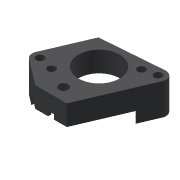
# Autodesk Inventor part: linact_top
Saved by Autodesk Inventor 2014 (Build 180170000, 170)
## iProperties
Created: 2015-04-17
Part Number: linact_top
Material: Generic
Document SubType Name: Modeling
Designer: Martin
Density: 1 g/cm^3
Appearance: Default
Mass: 1.23185 g
Surface Area: 12.9217 cm^2
Volume: 1.23185 cm^3
Author: Martin
Autodesk Inventor part; units mm, degrees
sketch "sk_mainbody" plane through (0, 0, 0) normal (0, 0, 1) x (1, 0, 0)
  line L0 (-7.1386, -0.6138) -> (9.4827, 3.383) construction
  line L1 (-10.6899, -8.9546) -> (-7.1386, -0.6138) projected
  arc A0 (-10.6899, -8.9546) -> (-10.0592, -11.3309) centre (-8.8497, -9.7381) ccw projected
  line L2 (-3.4497, -16.3498) -> (-10.0592, -11.3309) projected
  circle A1 centre (-8.8497, -9.7381) radius 1 projected
  circle A2 centre (9.9503, 1.4384) radius 1 projected
  arc A3 (11.7904, 0.655) -> (9.4827, 3.383) centre (9.9503, 1.4384) ccw projected
  line L3 (11.7904, 0.655) -> (4.5503, -16.3498) projected
  line L4 (4.5503, -16.3498) -> (-3.4497, -16.3498) projected
  circle A4 centre (0.5503, -4.1498) radius 3.4 construction
  circle A5 centre (0.5503, -13.1498) radius 1 construction
  circle A6 centre (0.5503, -4.1498) radius 5.25
  line L5 (-7.1386, -0.6138) -> (-5.9457, 2.1878)
  line L6 (-5.9457, 2.1878) -> (9.7927, 3.4322)
  circle A7 centre (0.5503, -13.1498) radius 1.2
  point P0 (0, 0)
  dimension "d0" = 10.5
  dimension "d1" = 9
  dimension "d37" = 2.4
  constraints: 4 end point, 2 centre point, 2 coincident, 1 parallel, 1 point on circle, 1 tangent
  measures "d0" diameter of A6
  measures "d1" angle of L0 L6
  measures "d37" diameter of A7
extrude "ext_mainbody" add sketch "sk_mainbody" along normal blind 5.2
sketch "sk_bottomsupport" plane through (0, 0, 0) normal (0, 0, 1) x (1, 0, 0)
  line L0 (-10.6899, -8.9546) -> (-7.1386, -0.6138) projected
  arc A0 (-10.6899, -8.9546) -> (-10.0592, -11.3309) centre (-8.8497, -9.7381) ccw projected
  line L1 (-3.4497, -16.3498) -> (-10.0592, -11.3309) projected
  line L2 (4.5503, -16.3498) -> (-3.4497, -16.3498) projected
  line L3 (11.7904, 0.655) -> (4.5503, -16.3498) projected
  arc A1 (11.7904, 0.655) -> (9.4827, 3.383) centre (9.9503, 1.4384) ccw projected
  line L4 (-7.1386, -0.6138) -> (9.4827, 3.383) projected
  circle A2 centre (-8.8497, -9.7381) radius 1 projected
  circle A3 centre (9.9503, 1.4384) radius 1 projected
  circle A4 centre (0.5503, -13.1498) radius 1 construction
  arc A5 (-6.417, -9.0187) -> (-7.5492, -13.2368) centre (0.5503, -13.1498) ccw
  circle A6 centre (-4.5247, -4.1498) radius 1 construction
  circle A7 centre (0.5503, -4.1498) radius 3.4 construction
  circle A8 centre (0.5503, -4.1498) radius 5 construction
  circle A9 centre (-5.0196, -10.6625) radius 2 construction
  circle A10 centre (6.5473, 0.6202) radius 2 construction
  circle A11 centre (6.5473, 0.6202) radius 1
  circle A12 centre (-5.0196, -10.6625) radius 1
  circle A13 centre (9.9503, 1.4384) radius 1.5 construction
  circle A14 centre (0.5503, -4.1498) radius 5.6627 construction
  arc A15 (-7.9094, -4.9768) -> (-6.417, -9.0187) centre (0.5503, -4.1498) ccw
  line L5 (-7.9094, -4.9768) -> (-8.8294, -4.5851)
  line L6 (8.0243, 3.0323) -> (8.4919, 1.0877)
  arc A16 (7.9873, -0.7678) -> (8.4919, 1.0877) centre (6.5473, 0.6202) ccw
  line L7 (-5.0196, -10.6625) -> (-7.1846, -13.5137) construction
  line L8 (-5.0196, -10.6625) -> (-2.8545, -7.8114) construction
  line L9 (7.9873, -0.7678) -> (9.7823, -4.0616)
  arc A17 (8.2936, -0.3548) -> (8.2887, -1.3207) centre (9.1667, -0.8422) ccw
  line L10 (9.7927, 3.4322) -> (-5.9457, 2.1878) projected
  line L11 (8.0243, 3.0323) -> (7.9629, 3.2876)
  point P0 (0, 0)
  point P1 (-5.2757, -0.1658)
  dimension "d12" = 10
  dimension "d16" = 3
  dimension "d5" = 8.1
  dimension "d13" = 4
  dimension "d15" = 2
  dimension "d17" = 11.3254
  dimension "d18" = 8.5
  dimension "d20" = 1
  dimension "d21" = 1
  dimension "d22" = 5.5
  constraints: 12 end point, 12 point on circle, 9 centre point, 8 point on line, 5 coincident, 5 tangent, 3 collinear, 3 equal radius, 3 perpendicular, 2 concentric, 7 other
  measures "d5" radius of A5
  measures "d13" diameter of A9
  measures "d15" diameter of A12
  measures "d17" diameter of A14
  measures "d18" radius of A15
  measures "d20" distance of L5.start L5.end
  measures "d21" radius of A17
  measures "d22" vertical distance of L9.end A1.centre
ref_plane "Work Plane1" through (-10.5497, -16.3498, -2.2) normal (0, 0, 1) x (1, 0, 0)
ref_plane "Work Plane2" through (-10.8497, -16.3498, -2.5) normal (0, 0, 1) x (1, 0, 0)
ref_plane "Work Plane3" through (-10.8497, -16.3498, -2.8) normal (0, 0, 1) x (1, 0, 0)
extrude "ext_bottomsupport" add sketch "sk_bottomsupport" against normal up to surface (2.8 mm away) contours L0 L5 A15 A5 L1 A0 | L11 L10 A1 L4 | L4 A1 L3 L9 A17 A16 L6
sketch "sk_mountholes" plane through (0, 0, 0) normal (0, 0, -1) x (-1, 0, 0)
  line L0 (-7.9629, 3.2876) -> (-8.4919, 1.0877) projected
  arc A0 (-8.4919, 1.0877) -> (-8.2936, -0.3548) centre (-6.5473, 0.6202) ccw projected
  line L1 (-9.7927, 3.4322) -> (5.9457, 2.1878) projected
  circle A1 centre (-6.5473, 0.6202) radius 2 projected
  circle A2 centre (5.0196, -10.6625) radius 2 projected
  circle A3 centre (-6.5473, 0.6202) radius 1 projected
  circle A4 centre (5.0196, -10.6625) radius 1 projected
  line L2 (-8.0243, 3.0323) -> (-7.9629, 3.2876) projected
  line L3 (-8.0243, 3.0323) -> (-8.4919, 1.0877) projected
  line L4 (-4.9629, 3.0503) -> (-5.0502, 1.9463)
  point P0 (0, 0)
  point P1 (-8.0383, 2.9491)
  dimension "d28" = 3
  constraints: 2 end point, 1 perpendicular, 1 point on circle, 1 point on line, 3 other
  measures "d28" horizontal distance of L4.start point (-7.963, 3.288)
extrude "ext_mountholes_head" cut sketch "sk_mountholes" against normal blind 3 contours L1 L4 A1 L0 | A1 A0 | A2 | A3 | A4
extrude "ext_mountholes_screw" cut sketch "sk_mountholes" against normal through all contours A3 | A4
sketch "Sketch8" plane through (0, 0, 0) normal (0, 0, -1) x (-1, 0, 0)
  line L0 (3.4497, -16.3498) -> (-4.5503, -16.3498) projected
  circle A0 centre (-0.5503, -13.1498) radius 1 projected
  circle A1 centre (-0.5503, -13.1498) radius 2.5
  line L1 (-0.5503, -13.1498) -> (-0.5503, -16.3498) construction
  line L2 (-1.3003, -15.5347) -> (-1.3003, -16.3498)
  line L3 (0.1997, -15.5347) -> (0.1997, -16.3498)
  point P0 (0, 0)
  dimension "d33" = 5
  dimension "d34" = 1.5
  constraints: 6 end point, 2 point on circle, 2 point on line, 1 centre point, 1 coincident, 1 midpoint, 1 perpendicular, 1 other
  measures "d33" diameter of A1
  measures "d34" distance between parallel lines of L3 L2
extrude "ext_gearhousing" cut sketch "Sketch8" against normal blind 1.2
equation "\"d37\" = general_dowel_diameter"
equation "\"general_dowel_diameter\" = 2.4"
body "Solid1"
